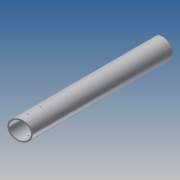
# Autodesk Inventor part: 2r2scs
Saved by Autodesk Inventor 2014 SP1 (Build 180222100, 222)
## iProperties
Company: HERA Project
Created: 2013-06-11
Part Number: 2r2scs
Material: PVC-Piping
Document SubType Name: Modeling
Designer: David DeBoer
Density: 1.4 g/cm^3
Description: spar cross support holder
Mass: 468.384 g
Surface Area: 1724.47 cm^2
Volume: 334.56 cm^3
Appearance: Smooth - White
Author: David DeBoer
Title: Hub-supporthold
Autodesk Inventor part; units mm, degrees
ref_plane "YZ Plane" through (0, 0, 0) normal (1, 0, 0) x (0, 1, 0)
ref_plane "XZ Plane" through (0, 0, 0) normal (0, 1, 0) x (-1, 0, 0)
ref_plane "XY Plane" through (0, 0, 0) normal (0, 0, 1) x (1, 0, 0)
sketch "Sketch1" plane through (0, 0, 0) normal (0, 0, 1) x (1, 0, 0)
  circle A0 centre (0, 0) radius 30.1625
  circle A1 centre (0, 0) radius 26.2509
  dimension "d0" = 60.325
  dimension "d2" = 3.9116
  constraints: 2 centre point, 1 coincident
  measures "d0" diameter of A0
  measures "d2" radial gap between concentric circles of A1 A0
extrude "Extrusion1" add sketch "Sketch1" along normal blind 440
sketch "Sketch18" plane through (0, 0, 440) normal (0, 0, 1) x (1, 0, 0)
  circle A0 centre (0, 0) radius 26.2509 projected
  circle A1 centre (0, 0) radius 30.1625 projected
  point P0 (-30.1625, 0)
  constraints: 1 horizontal alignment, 1 other
ref_plane "Work Plane9" through (-30.1625, 0, 440) normal (0.258819, 0, 0.9659258) x (0, 1, 0)
sketch "Sketch19" plane through (-30.1625, 0, 440) normal (0.258819, 0, 0.9659258) x (0, 1, 0)
  line L0 (-31.6137, -94.9476) -> (64.4261, -94.9476)
  line L1 (64.4261, -94.9476) -> (64.4261, 6.6524)
  line L2 (64.4261, 6.6524) -> (-31.6137, 6.6524)
  line L3 (-31.6137, 6.6524) -> (-31.6137, -94.9476)
  point P0 (0, -143.0151)
  dimension "d61" = 101.6
  constraints: 8 end point, 2 parallel, 1 horizontal, 1 perpendicular
  measures "d61" distance of L2.end L0.start
extrude "Extrusion11" cut sketch "Sketch19" along normal blind 25.4
sketch "Sketch20" plane through (0, 0, 0) normal (0, 0, -1) x (-1, 0, 0)
  circle A0 centre (0, 0) radius 26.2509 projected
  circle A1 centre (0, 0) radius 30.1625 projected
  point P0 (0, 30.1625)
  point P1 (0, -30.1625)
  constraints: 2 point on circle
ref_plane "Work Plane10" through (0, 30.1625, 0) normal (0, 1, 0) x (-1, 0, 0)
ref_plane "Work Plane11" through (0, -30.1625, 0) normal (0, -1, 0) x (1, 0, 0)
sketch "Sketch21" plane through (0, 30.1625, 0) normal (0, 1, 0) x (-1, 0, 0)
  line L0 (-3.1444, 432.8221) -> (3.2056, 432.8221)
  line L1 (3.2056, 432.8221) -> (3.2056, 331.2221)
  line L2 (3.2056, 331.2221) -> (-3.1444, 331.2221)
  line L3 (-3.1444, 331.2221) -> (-3.1444, 432.8221)
  line L4 (0.0306, 432.8221) -> (0.0306, 331.2221) construction
  point P0 (0, 0)
  dimension "d64" = 6.35
  dimension "d65" = 101.6
  constraints: 10 end point, 2 midpoint, 2 parallel, 1 horizontal, 1 perpendicular
  measures "d64" distance of L1.end L2.end
  measures "d65" distance of L0.end L1.end
extrude "flat1" cut sketch "Sketch21" against normal blind 0.254
sketch "Sketch22" plane through (0, -30.1625, 0) normal (0, -1, 0) x (1, 0, 0)
  line L0 (-3.1568, 331.2379) -> (3.1932, 331.2379)
  line L1 (3.1932, 331.2379) -> (3.1932, 432.8379)
  line L2 (3.1932, 432.8379) -> (-3.1568, 432.8379)
  line L3 (-3.1568, 432.8379) -> (-3.1568, 331.2379)
  line L4 (0.0182, 432.8379) -> (0.0182, 331.2379) construction
  point P0 (0, 0)
  dimension "d68" = 6.35
  dimension "d69" = 101.6
  constraints: 10 end point, 2 midpoint, 2 parallel, 1 horizontal, 1 perpendicular
  measures "d68" distance of L0.start L0.end
  measures "d69" distance of L2.end L0.start
extrude "flat2" cut sketch "Sketch22" against normal blind 0.254
sketch "Sketch23" plane through (0, -29.9085, 0) normal (0, -1, 0) x (1, 0, 0)
  circle A0 centre (0, 407.3638) radius 1.4603
  circle A1 centre (0, 369.2638) radius 1.4603
  point P0 (-3.1568, 432.7638)
  point P1 (0, 0)
  dimension "d73" = 38.1
  dimension "d74" = 25.4
  constraints: 2 centre point
  measures "d73" distance of A0.centre A1.centre
  measures "d74" vertical distance of point (-3.157, 432.764) A0.centre
hole "Hole1" at (0, -29.9085, 407.3638) at (0, -29.9085, 369.2638) direction (0, 1, 0) diameter 3.175 end through all
body "Solid1"
